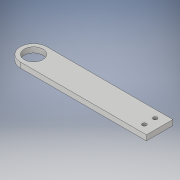
# Autodesk Inventor part: TapeMeasureBracketSide
Saved by Autodesk Inventor 2019 (Build 230136000, 136)
## iProperties
Created: 2018-11-04
Part Number: TapeMeasureBracketSide
Material: Generic
Document SubType Name: Modeling
Designer: mrhftc
Density: 1 g/cm^3
Appearance: Default
Author: mrhftc
Autodesk Inventor part; units mm, degrees
ref_plane "YZ Plane" through (0, 0, 0) normal (1, 0, 0) x (0, 1, 0)
ref_plane "XZ Plane" through (0, 0, 0) normal (0, 1, 0) x (-1, 0, 0)
ref_plane "XY Plane" through (0, 0, 0) normal (0, 0, 1) x (1, 0, 0)
sketch "Sketch1" plane through (0, 0, 0) normal (0, 1, 0) x (-1, 0, 0)
  line L0 (-47.625, 10) -> (47.625, 10)
  line L1 (47.625, -10) -> (-47.625, -10)
  line L2 (-47.625, -10) -> (-47.625, 10)
  line L3 (-47.625, 10) -> (47.625, -10) construction
  line L4 (47.625, 10) -> (-47.625, -10) construction
  circle A0 centre (47.625, 0) radius 7
  arc A1 (47.625, -10) -> (47.625, 10) centre (47.625, 0) ccw
  circle A2 centre (-40.125, 4.1) radius 1.5
  line L5 (-38.625, 0) -> (-49.4241, 0)
  circle A3 centre (-40.125, -4.1) radius 1.5
  point P0 (0, 0)
  dimension "d3" = 14
  dimension "d4" = 95.25
  dimension "d5" = 20
  dimension "d6" = 3
  dimension "d7" = 7.5
  dimension "d9" = 5.9
  dimension "d10" = 8.2
  constraints: 12 end point, 4 centre point, 2 midpoint, 2 point on circle, 1 coincident, 1 horizontal, 1 parallel, 1 perpendicular, 1 symmetric about line, 1 other
  measures "d3" diameter of A0
  measures "d4" distance from line of L2 A0.centre
  measures "d5" distance of L1.end L0.start
  measures "d6" diameter of A2
  measures "d7" distance from line of A2.centre L2
  measures "d9" distance from line of L0 A2.centre
  measures "d10" distance of A2.centre A3.centre
extrude "Extrusion1" add sketch "Sketch1" along normal blind 4
body "Solid1"
